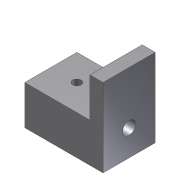
# Autodesk Inventor part: ArmPivotBlock
Saved by Autodesk Inventor 2012 (Build 160160000, 160)
## iProperties
Created: 2013-01-19
Part Number: ArmPivotBlock
Material: Default
Document SubType Name: Modeling
Designer: JesseK
Density: 1 g/cm^3
Mass: 20.126 g
Surface Area: 63.8063 cm^2
Volume: 20.126 cm^3
Author: JesseK
Autodesk Inventor part; units mm, degrees
ref_plane "YZ Plane" through (0, 0, 0) normal (1, 0, 0) x (0, 1, 0)
ref_plane "XZ Plane" through (0, 0, 0) normal (0, 1, 0) x (-1, 0, 0)
ref_plane "XY Plane" through (0, 0, 0) normal (0, 0, 1) x (1, 0, 0)
sketch "Sketch1" plane through (0, 0, 0) normal (0, 0, 1) x (1, 0, 0)
  line L0 (0, 0) -> (38.1, 0)
  line L1 (38.1, 0) -> (38.1, 38.1)
  line L2 (38.1, 38.1) -> (0, 38.1)
  line L3 (0, 38.1) -> (0, 0)
  dimension "d0" = 38.1
  dimension "d1" = 38.1
  constraints: 8 end point, 2 parallel, 1 horizontal, 1 perpendicular
  measures "d0" distance of L2.end L0.start
  measures "d1" distance of L1.end L2.end
extrude "Extrusion1" add sketch "Sketch1" along normal blind 25.4
sketch "Sketch2" plane through (38.1, 0, 0) normal (1, 0, 0) x (0, 0, -1)
  line L0 (0, 0) -> (0, 38.1) projected
  circle A0 centre (-12.7, 12.7) radius 3.175
  line L1 (0, 0) -> (-25.4, 0) projected
  dimension "d5" = 12.7
  dimension "d6" = 6.35
  dimension "d18" = 12.7
  constraints: 1 centre point
  measures "d5" distance from line of L0 A0.centre
  measures "d6" diameter of A0
  measures "d18" distance from line of L1 A0.centre
extrude "Extrusion2" cut sketch "Sketch2" against normal through all
sketch "Sketch3" plane through (0, 0, 25.4) normal (0, 0, 1) x (1, 0, 0)
  line L0 (38.1, 38.1) -> (38.1, 0) projected
  line L1 (0, 38.1) -> (38.1, 38.1) projected
  line L2 (0, 38.1) -> (31.75, 38.1)
  line L3 (31.75, 38.1) -> (31.75, 19.05)
  line L4 (31.75, 19.05) -> (0, 19.05)
  line L5 (0, 19.05) -> (0, 38.1)
  dimension "d10" = 19.05
  dimension "d19" = 6.35
  constraints: 8 end point, 2 parallel, 1 horizontal, 1 perpendicular
  measures "d10" distance between parallel lines of L1 L4
  measures "d19" distance between parallel lines of L0 L3
extrude "Extrusion3" cut sketch "Sketch3" against normal through all
sketch "Sketch5" plane through (0, 0, 0) normal (0, -1, 0) x (1, 0, 0)
  line L0 (38.1, 25.4) -> (0, 25.4) projected
  line L1 (0, 0) -> (0, 25.4) projected
  circle A0 centre (12.7, 12.7) radius 2.0735
  dimension "d20" = 12.7
  dimension "d21" = 12.7
  constraints: 1 centre point
  measures "d20" distance from line of L0 A0.centre
  measures "d21" distance from line of L1 A0.centre
extrude "Extrusion5" cut sketch "Sketch5" against normal through all
body "Solid1"
